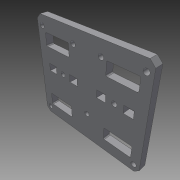
# Autodesk Inventor part: x_carryage_back
Saved by Autodesk Inventor 2014 (Build 180170000, 170)
## iProperties
Created: 2014-03-27
Part Number: x_carryage_back
Material: Plywood, Finish
Document SubType Name: Modeling
Designer: buben
Density: 0.552 g/cm^3
Appearance: Plywood - New
Author: buben
Autodesk Inventor part; units mm, degrees
ref_plane "YZ Plane" through (0, 0, 0) normal (1, 0, 0) x (0, 1, 0)
ref_plane "XZ Plane" through (0, 0, 0) normal (0, 1, 0) x (-1, 0, 0)
ref_plane "XY Plane" through (0, 0, 0) normal (0, 0, 1) x (1, 0, 0)
sketch "Sketch1" plane through (0, 0, 0) normal (0, 1, 0) x (-1, 0, 0)
  line L0 (0, 0) -> (-100, 0)
  line L1 (-100, 0) -> (-100, -88)
  line L2 (-100, -88) -> (0, -88)
  line L3 (0, -88) -> (0, 0)
  line L4 (-9, -23.5) -> (-32, -23.5)
  line L5 (-33, -22.5) -> (-33, -13.5)
  line L6 (-32, -12.5) -> (-9, -12.5)
  line L7 (-8, -13.5) -> (-8, -22.5)
  arc A0 (-9, -23.5) -> (-8, -22.5) centre (-9, -22.5) ccw
  arc A1 (-8, -13.5) -> (-9, -12.5) centre (-9, -13.5) ccw
  arc A2 (-32, -12.5) -> (-33, -13.5) centre (-32, -13.5) ccw
  arc A3 (-33, -22.5) -> (-32, -23.5) centre (-32, -22.5) ccw
  line L8 (-9, -77.5) -> (-32, -77.5)
  line L9 (-33, -76.5) -> (-33, -67.5)
  line L10 (-32, -66.5) -> (-9, -66.5)
  line L11 (-8, -67.5) -> (-8, -76.5)
  arc A4 (-9, -77.5) -> (-8, -76.5) centre (-9, -76.5) ccw
  arc A5 (-8, -67.5) -> (-9, -66.5) centre (-9, -67.5) ccw
  arc A6 (-32, -66.5) -> (-33, -67.5) centre (-32, -67.5) ccw
  arc A7 (-33, -76.5) -> (-32, -77.5) centre (-32, -76.5) ccw
  line L12 (-68, -77.5) -> (-91, -77.5)
  line L13 (-92, -76.5) -> (-92, -67.5)
  line L14 (-91, -66.5) -> (-68, -66.5)
  line L15 (-67, -67.5) -> (-67, -76.5)
  arc A8 (-68, -77.5) -> (-67, -76.5) centre (-68, -76.5) ccw
  arc A9 (-67, -67.5) -> (-68, -66.5) centre (-68, -67.5) ccw
  arc A10 (-91, -66.5) -> (-92, -67.5) centre (-91, -67.5) ccw
  arc A11 (-92, -76.5) -> (-91, -77.5) centre (-91, -76.5) ccw
  line L16 (-68, -23.5) -> (-91, -23.5)
  line L17 (-92, -22.5) -> (-92, -13.5)
  line L18 (-91, -12.5) -> (-68, -12.5)
  line L19 (-67, -13.5) -> (-67, -22.5)
  arc A12 (-68, -23.5) -> (-67, -22.5) centre (-68, -22.5) ccw
  arc A13 (-67, -13.5) -> (-68, -12.5) centre (-68, -13.5) ccw
  arc A14 (-91, -12.5) -> (-92, -13.5) centre (-91, -13.5) ccw
  arc A15 (-92, -22.5) -> (-91, -23.5) centre (-91, -22.5) ccw
  line L20 (-8, -72) -> (-92, -72) construction
  line L21 (-92, -18) -> (-8, -18) construction
  point P0 (-50, -18)
  point P1 (-50, 0)
  dimension "d0" = 100
  dimension "d1" = 88
  dimension "d2" = 1
  dimension "d3" = 25
  dimension "d4" = 11
  dimension "d5" = 1
  dimension "d6" = 25
  dimension "d7" = 11
  dimension "d8" = 1
  dimension "d9" = 25
  dimension "d10" = 11
  dimension "d11" = 1
  dimension "d12" = 25
  dimension "d13" = 11
  dimension "d14" = 54
  dimension "d15" = 18
  dimension "d16" = 8
  constraints: 44 end point, 32 point on circle, 32 tangent, 16 centre point, 12 equal radius, 10 parallel, 6 midpoint, 5 horizontal, 5 perpendicular, 4 collinear, 1 vertical alignment
  measures "d0" distance of L0.start L0.end
  measures "d1" distance of L2.end L0.start
  measures "d2" radius of A0
  measures "d3" distance between parallel lines of L7 L5
  measures "d4" distance between parallel lines of L6 L4
  measures "d5" radius of A4
  measures "d6" distance between parallel lines of L11 L9
  measures "d7" distance between parallel lines of L10 L8
  measures "d8" radius of A8
  measures "d9" distance between parallel lines of L15 L13
  measures "d10" distance between parallel lines of L14 L12
  measures "d11" radius of A12
  measures "d12" distance between parallel lines of L19 L17
  measures "d13" distance between parallel lines of L18 L16
  measures "d14" distance of L20.start L21.end
  measures "d15" distance from line of L0 L21.end
  measures "d16" distance between parallel lines of L1 L13
extrude "Extrusion1" add sketch "Sketch1" along normal blind 6.5
chamfer "Chamfer1" distance 4 angle 45 4 edges at (0, 3.25, 0) (100, 3.25, 0) (100, 3.25, -88) (0, 3.25, -88)
sketch "Sketch2" plane through (0, 6.5, 0) normal (0, 1, 0) x (1, 0, 0)
  line L0 (4, 0) -> (96, 0) projected
  line L1 (9.5, 44) -> (17.5, 44)
  line L2 (17.5, 44) -> (17.5, 37.5)
  line L3 (17.5, 37.5) -> (9.5, 37.5)
  line L4 (9.5, 37.5) -> (9.5, 44)
  line L5 (32.5, 44) -> (40.5, 44)
  line L6 (40.5, 44) -> (40.5, 37.5)
  line L7 (40.5, 37.5) -> (32.5, 37.5)
  line L8 (32.5, 37.5) -> (32.5, 44)
  line L9 (59.5, 44) -> (67.5, 44)
  line L10 (67.5, 44) -> (67.5, 37.5)
  line L11 (67.5, 37.5) -> (59.5, 37.5)
  line L12 (59.5, 37.5) -> (59.5, 44)
  line L13 (82.5, 44) -> (90.5, 44)
  line L14 (90.5, 44) -> (90.5, 37.5)
  line L15 (90.5, 37.5) -> (82.5, 37.5)
  line L16 (82.5, 37.5) -> (82.5, 44)
  line L17 (17.5, 44) -> (32.5, 37.5) construction
  line L18 (32.5, 44) -> (17.5, 37.5) construction
  line L19 (67.5, 37.5) -> (82.5, 44) construction
  line L20 (82.5, 37.5) -> (67.5, 44) construction
  circle A0 centre (25, 40.75) radius 2.25
  circle A1 centre (75, 40.75) radius 2.25
  line L21 (40.5, 40.75) -> (59.5, 40.75) construction
  point P0 (0, 0)
  point P1 (50, 40.75)
  point P2 (50, 0)
  dimension "d22" = 6.5
  dimension "d23" = 8
  dimension "d24" = 15
  dimension "d25" = 15
  dimension "d26" = 4.5
  dimension "d27" = 4.5
  dimension "d28" = 50
  dimension "d29" = 37.5
  constraints: 42 end point, 9 collinear, 8 parallel, 6 midpoint, 4 horizontal, 4 perpendicular, 2 centre point, 1 vertical alignment
  measures "d22" distance of L3.end L1.start
  measures "d23" distance of L1.start L1.end
  measures "d24" distance between parallel lines of L8 L2
  measures "d25" distance between parallel lines of L16 L10
  measures "d26" diameter of A1
  measures "d27" diameter of A0
  measures "d28" distance of A1.centre A0.centre
  measures "d29" distance between parallel lines of L0 L3
extrude "Extrusion2" cut sketch "Sketch2" against normal through all
sketch "Sketch3" plane through (0, 6.5, 0) normal (0, 1, 0) x (1, 0, 0)
  line L0 (9, 77.5) -> (32, 77.5) projected
  line L1 (8, 67.5) -> (8, 76.5) projected
  line L2 (32, 12.5) -> (9, 12.5) projected
  line L3 (0, 84) -> (0, 4) projected
  line L4 (4, 0) -> (96, 0) projected
  line L5 (100, 4) -> (100, 84) projected
  line L6 (5, 81.75) -> (95, 81.75) construction
  line L7 (95, 81.75) -> (95, 8.25) construction
  line L8 (95, 8.25) -> (5, 8.25) construction
  line L9 (5, 8.25) -> (5, 81.75) construction
  circle A0 centre (5, 81.75) radius 4.5 construction
  circle A1 centre (95, 81.75) radius 4.5 construction
  circle A2 centre (95, 8.25) radius 4.5 construction
  circle A3 centre (5, 8.25) radius 4.5 construction
  circle A4 centre (5, 81.75) radius 2.25
  circle A5 centre (95, 81.75) radius 2.25
  circle A6 centre (95, 8.25) radius 2.25
  circle A7 centre (5, 8.25) radius 2.25
  point P0 (0, 0)
  dimension "d32" = 9
  dimension "d33" = 4.5
  dimension "d34" = 8
  dimension "d35" = 12.5
  dimension "d36" = 5
  dimension "d37" = 5
  dimension "d38" = 8.25
  dimension "d39" = 4.25
  constraints: 8 centre point, 8 coincident, 8 end point, 6 equal radius, 2 parallel, 1 horizontal, 1 perpendicular
  measures "d32" diameter of A0
  measures "d33" diameter of A4
  measures "d34" distance between parallel lines of L3 L1
  measures "d35" distance between parallel lines of L4 L2
  measures "d36" distance between parallel lines of L3 L9
  measures "d37" distance between parallel lines of L5 L7
  measures "d38" distance between parallel lines of L4 L8
  measures "d39" distance between parallel lines of L0 L6
extrude "Extrusion3" cut sketch "Sketch3" against normal through all
sketch "Sketch4" plane through (0, 6.5, 0) normal (0, 1, 0) x (1, 0, 0)
  line L0 (4, 0) -> (96, 0) projected
  line L1 (96, 88) -> (4, 88) projected
  circle A0 centre (37.5, 11.75) radius 2.25
  circle A1 centre (62.5, 11.75) radius 2.25
  line L2 (37.5, 11.75) -> (62.5, 11.75) construction
  point P0 (0, 0)
  point P1 (50, 11.75)
  point P2 (50, 0)
  dimension "d42" = 4.5
  dimension "d43" = 25
  dimension "d44" = 11.75
  constraints: 2 centre point, 2 end point, 2 midpoint, 1 equal radius, 1 horizontal alignment, 1 parallel, 1 vertical alignment
  measures "d42" diameter of A0
  measures "d43" distance of L2.start L2.end
  measures "d44" distance between parallel lines of L0 L2
extrude "Extrusion4" cut sketch "Sketch4" against normal through all
sketch "Sketch5" plane through (0, 6.5, 0) normal (0, 1, 0) x (1, 0, 0)
  line L0 (32.5, 44) -> (40.5, 44) projected
  line L1 (96, 88) -> (4, 88) projected
  circle A0 centre (50, 63.75) radius 2.25
  point P0 (0, 0)
  point P1 (50, 88)
  dimension "d47" = 4.5
  dimension "d48" = 19.75
  constraints: 1 centre point, 1 midpoint, 1 vertical alignment
  measures "d47" diameter of A0
  measures "d48" distance from line of L0 A0.centre
extrude "Extrusion5" cut sketch "Sketch5" against normal through all
equation "\"d25\" = d24"
equation "\"d37\" = d36"
equation "\"d39\" = d35 - d38"
body "Solid1"
